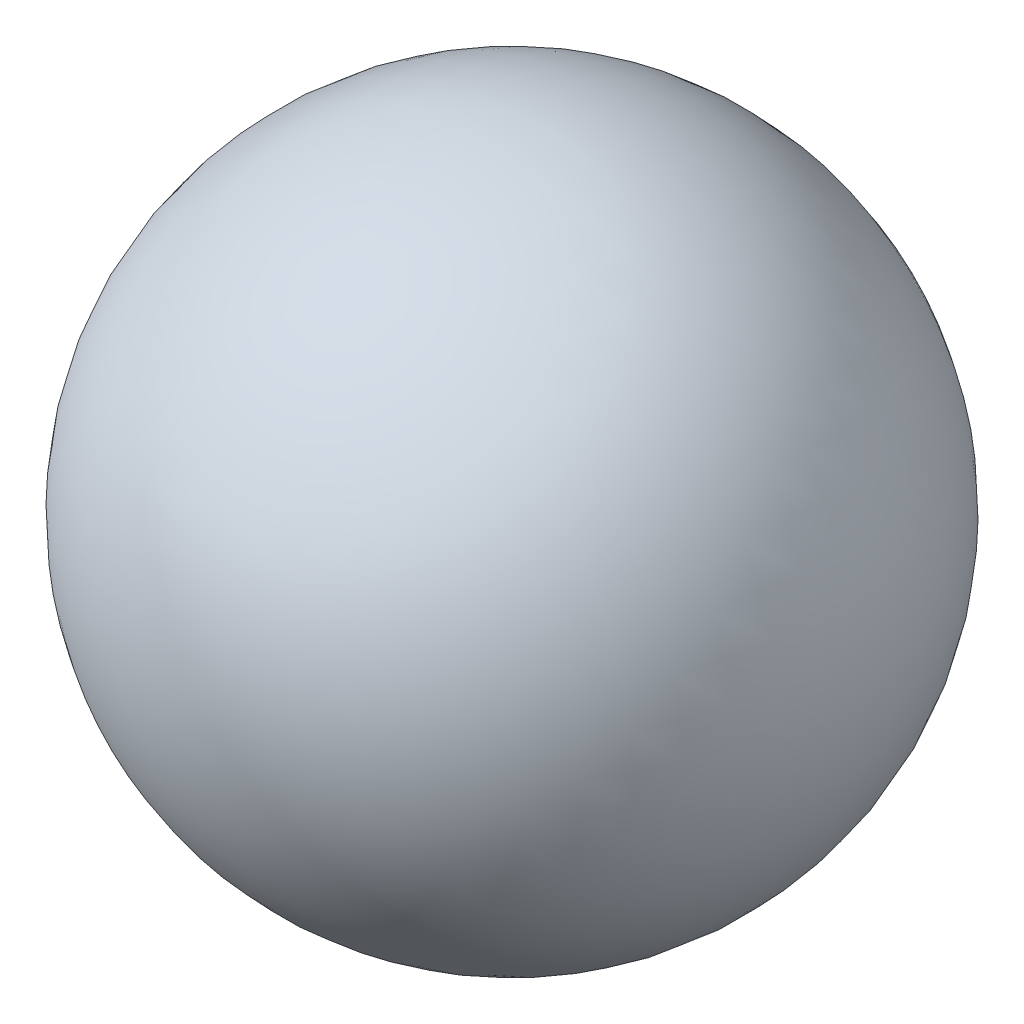
# Autodesk Inventor part: ucfl-IEC_BBY_006-25-34--52-15-39-7.938
Saved by Autodesk Inventor 2019 (Build 230136000, 136)
## iProperties
Created: 2024-04-15
Part Number: ucfl-IEC_BBY_006-25-34--52-15-39-7.938
Material: Generic
Catalog Web Link: www.cadenas.de
Description: ayf_002hc_hh_hy_ball-Oval flanged housings for Y-bearings
Vendor: SKF
Document SubType Name: Modeling
Designer: psAdmin
Manufacturer: SKF
Mass: 0.261898 g
Surface Area: 1.97958 cm^2
Volume: 0.261898 cm^3
Density: 1 g/cm^3
Appearance: PSOLRGB-255-255-0
Category: PARTsolutions
Company: SKF
Title: ucfl-IEC_BBY_006-25-34--52-15-39-7.938
Author: Cadenas PARTsolutions
Comments: Oval flanged housings for Y-bearings
PSOL_IDENT_0: {$CADENAS_DATA/23d-libs/skf/bearings_units_and_housings/bearing_units/ball_bearing_units/y-units/y-b
PSOL_IDENT_1: earing_oval_flanged_units_parts/ayf_002hc_hh_hy_ayd_001hp_ball.prj},232 {VTYP=3D},{NB=ucfl-IEC_BBY_0
PSOL_IDENT_2: 06-25-34--52-15-39-7.938},{LINA=ucfl-IEC_BBY_006-25-34--52-15-39-7.938},{NN=ayf_002hc_hh_hy_ball},{D
PSOL_IDENT_3: ATE=28.11.2022 11:15:05},{GEOMDATE=24.11.2022 12:11:15},{VERSION=},{LINEID=9310},{WBVAR=},{WBNUMERIC=
PSOL_IDENT_4: }  {NB=ucfl-IEC_BBY_006-25-34--52-15-39-7.938},{LINA=ucfl-IEC_BBY_006-25-34--52-15-39-7.938},{KT=DUM
PSOL_IDENT_5: MY},{DD=25.0000},{D=52},{B=34.000},{C=15.000},{PITCH=39.000},{DW=7.938},{FO=IEC_BBY_006},{DESIGN=ucf
PSOL_IDENT_6: l},{X=0},{PN=}
NB: ucfl-IEC_BBY_006-25-34--52-15-39-7.938
NN: ayf_002hc_hh_hy_ball
NT: Oval flanged housings for Y-bearings
NBSYN: $DESIGN.-$FO.-$DD.-$B.-$PN.-$D.-$C.-$PITCH.-$DW.
LINA: ucfl-IEC_BBY_006-25-34--52-15-39-7.938
CATALOG: SKF
B: 34
C: 15
PITCH: 39
DW: 7.938
FO: IEC_BBY_006
X: 0
SUPPLIER: SKF
ARTICLENO: ucfl-IEC_BBY_006-25-34--52-15-39-7.938
BOMINFO: ucfl-IEC_BBY_006-25-34--52-15-39-7.938
CREATOR: CADENAS GmbH
Autodesk Inventor part; units mm, degrees
sketch "Sketch_11" plane through (0, 0, 0) normal (0, 0, 1) x (1, 0, 0)
  line L0 (3.969, 19.5) -> (-3.969, 19.5)
  arc A0 (3.969, 19.5) -> (-3.969, 19.5) centre (0, 19.5) ccw
  line L1 (3.969, 19.5) -> (-3.969, 19.5)
  constraints: 4 end point, 2 point on circle, 1 centre point
revolve "Revolution1" add sketch "Sketch_11" angle 360 about axis through (3.969, 19.5, 0) along (1, 0, 0)
ref_plane "ball_XY" through (0, 19.5, 0) normal (1, 0, 0) x (0, 0, -1)
ref_plane "ball_YZ" through (0, 19.5, 0) normal (0, 0, -1) x (0, 1, 0)
ref_plane "ball_ZX" through (0, 19.5, 0) normal (0, 1, 0) x (1, 0, 0)
body "Solid1"
